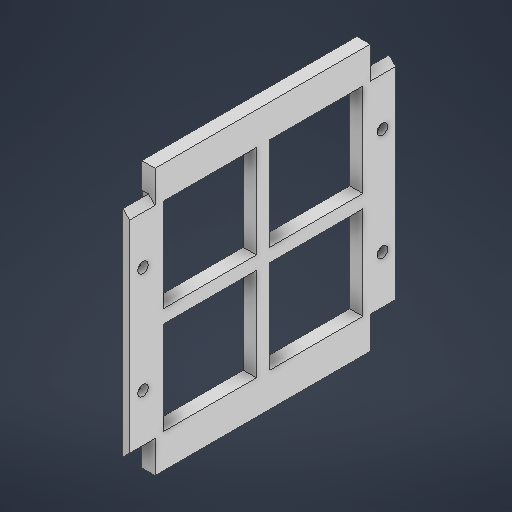
# Autodesk Inventor part: Side Panel
Saved by Autodesk Inventor 2026.1 (Build 301233020, 233B)
## iProperties
Created: 2025-10-16
Part Number: Side Panel
Material: Generic
Document SubType Name: Modeling
Designer: scott
Density: 1 g/cm^3
Appearance: Default
Author: scott
Autodesk Inventor part; units mm, degrees
ref_plane "YZ Plane" through (0, 0, 0) normal (1, 0, 0) x (0, 1, 0)
ref_plane "XZ Plane" through (0, 0, 0) normal (0, 1, 0) x (-1, 0, 0)
ref_plane "XY Plane" through (0, 0, 0) normal (0, 0, 1) x (1, 0, 0)
sketch "Sketch1" plane through (0, 0, 0) normal (1, 0, 0) x (0, 1, 0)
  line L0 (-40.43, 50) -> (40.43, 50)
  line L1 (50, 40.43) -> (50, -40.43)
  line L2 (40.43, -50) -> (-40.43, -50)
  line L3 (-50, -40.43) -> (-50, 40.43)
  line L4 (40.43, 50) -> (40.43, 40.43)
  line L5 (40.43, 40.43) -> (50, 40.43)
  line L6 (-50, 40.43) -> (-40.43, 40.43)
  line L7 (-40.43, 40.43) -> (-40.43, 50)
  line L8 (-40.43, -50) -> (-40.43, -40.43)
  line L9 (-40.43, -40.43) -> (-50, -40.43)
  line L10 (50, -40.43) -> (40.43, -40.43)
  line L11 (40.43, -40.43) -> (40.43, -50)
  line L12 (2.75, 2.3115) -> (37.75, 2.3115)
  line L13 (37.75, 2.3115) -> (37.75, 37.3115)
  line L14 (37.75, 37.3115) -> (2.75, 37.3115)
  line L15 (2.75, 37.3115) -> (2.75, 2.3115)
  line L16 (2.75, -37.6885) -> (37.75, -37.6885)
  line L17 (2.75, -2.6885) -> (2.75, -37.6885)
  line L18 (37.75, -2.6885) -> (2.75, -2.6885)
  line L19 (37.75, -37.6885) -> (37.75, -2.6885)
  line L20 (-37.25, 2.3115) -> (-2.25, 2.3115)
  line L21 (-37.25, 37.3115) -> (-37.25, 2.3115)
  line L22 (-2.25, 37.3115) -> (-37.25, 37.3115)
  line L23 (-2.25, 2.3115) -> (-2.25, 37.3115)
  line L24 (-37.25, -37.6885) -> (-2.25, -37.6885)
  line L25 (-37.25, -2.6885) -> (-37.25, -37.6885)
  line L26 (-2.25, -2.6885) -> (-37.25, -2.6885)
  line L27 (-2.25, -37.6885) -> (-2.25, -2.6885)
  line L28 (40.43, 40.43) -> (50, 40.43)
  line L29 (50, 40.43) -> (50, 50)
  line L30 (50, 50) -> (40.43, 50)
  line L31 (40.43, 50) -> (40.43, 40.43)
  line L32 (40.43, -40.43) -> (50, -40.43)
  line L33 (50, -40.43) -> (50, -50)
  line L34 (50, -50) -> (40.43, -50)
  line L35 (40.43, -50) -> (40.43, -40.43)
  line L36 (-40.43, -40.43) -> (-50, -40.43)
  line L37 (-50, -40.43) -> (-50, -50)
  line L38 (-50, -50) -> (-40.43, -50)
  line L39 (-40.43, -50) -> (-40.43, -40.43)
  line L40 (-40.43, 40.43) -> (-50, 40.43)
  line L41 (-50, 40.43) -> (-50, 50)
  line L42 (-50, 50) -> (-40.43, 50)
  line L43 (-40.43, 50) -> (-40.43, 40.43)
  circle A0 centre (20.0008, 45) radius 2
  circle A1 centre (20.0008, -45) radius 2
  circle A2 centre (-19.9992, 45) radius 2
  circle A3 centre (-19.9992, -45) radius 2
  point P0 (0, 0)
  point P1 (50, 45.215)
  dimension "d7" = 9.57
  dimension "d8" = 9.57
  dimension "d11" = 360
  dimension "d13" = 80.86
  dimension "d14" = 100
  dimension "d15" = 35
  dimension "d16" = 35
  dimension "d19" = 40
  dimension "d22" = 40
  dimension "d25" = 4
  dimension "d26" = 30
  dimension "d27" = 5
  dimension "d30" = 90
  dimension "d33" = 40
  dimension "d36" = 12.25
  constraints: 88 end point, 12 parallel, 8 horizontal, 6 perpendicular, 4 centre point, 3 point on line, 2 vertical, 1 midpoint, 51 other
  measures "d7" distance of L1.start L4.end
  measures "d8" distance of L0.end L4.end
  measures "d13" distance of L1.end L1.start
  measures "d14" distance of L3.start L1.end
  measures "d15" distance of L14.end L13.end
  measures "d16" distance of L13.end L12.end
  measures "d19" distance of L12.start L16.start
  measures "d22" distance of L12.start L20.start
  measures "d25" diameter of A0
  measures "d26" distance of A0.centre point (50, 45.215)
  measures "d27" distance from line of A0.centre L0
  measures "d30" distance of A0.centre A1.centre
  measures "d33" distance of A0.centre A2.centre
  measures "d36" distance between parallel lines of L13 L1
extrude "Extrusion1" add sketch "Sketch1" along normal blind 5 contours L0 L4 L5 L1 L10 L11 L2 L8 L9 L3 L6 L7
sketch "Sketch2" plane through (0, -40.43, 50) normal (0, 0, 1) x (1, 0, 0)
  line L0 (0, -9.57) -> (0, 0) projected
  line L1 (0, 80.86) -> (5, 80.86) projected
  line L2 (0, 0) -> (2.5, 0)
  line L3 (2.5, 0) -> (2.5, 80.86)
  line L4 (2.5, 80.86) -> (0, 80.86)
  line L5 (0, 80.86) -> (0, 0)
  point P0 (0, 40.43)
  constraints: 8 end point, 2 parallel, 1 horizontal, 1 midpoint, 1 perpendicular
extrude "Extrusion2" cut sketch "Sketch2" against normal blind 10
sketch "Sketch3" plane through (0, -40.43, -50) normal (0, 0, -1) x (-1, 0, 0)
  line L0 (-2.5, 80.86) -> (-2.5, 0) projected
  line L1 (0, 0) -> (-2.5, 0)
  line L2 (-2.5, 0) -> (-2.5, 80.86)
  line L3 (-2.5, 80.86) -> (0, 80.86)
  line L4 (0, 80.86) -> (0, 0)
  point P0 (0, 40.43)
  constraints: 8 end point, 2 parallel, 1 horizontal, 1 perpendicular
extrude "Extrusion3" cut sketch "Sketch3" against normal blind 10
chamfer "Chamfer3" distance 2.5 angle 45 4 edges at (5, -40.43, 45.215) (5, 40.43, 45.215) (5, -40.43, -45.215) (5, 40.43, -45.215)
body "Solid1"
